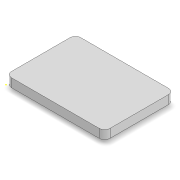
# Autodesk Inventor part: Gyro_box_Top
Saved by Autodesk Inventor 2020 (Build 240168000, 168)
## iProperties
Created: 2019-08-08
Part Number: Gyro_box_Top
Material: Generic
Document SubType Name: Modeling
Designer: chitl
Density: 1 g/cm^3
Appearance: Default
Author: chitl
Autodesk Inventor part; units mm, degrees
ref_plane "YZ Plane" through (0, 0, 0) normal (1, 0, 0) x (0, 1, 0)
ref_plane "XZ Plane" through (0, 0, 0) normal (0, 1, 0) x (-1, 0, 0)
ref_plane "XY Plane" through (0, 0, 0) normal (0, 0, 1) x (1, 0, 0)
sketch "Sketch1" plane through (0, 0, 0) normal (0, 1, 0) x (-1, 0, 0)
  line L0 (0, 0) -> (-56.9976, 0)
  line L1 (-56.9976, 0) -> (-56.9976, -40.1066)
  line L2 (-56.9976, -40.1066) -> (0, -40.1066)
  line L3 (0, -40.1066) -> (0, 0)
  dimension "d0" = 40.1066
  dimension "d1" = 56.9976
  constraints: 8 end point, 2 parallel, 1 horizontal, 1 perpendicular
  measures "d0" distance of L2.end L0.start
  measures "d1" distance between parallel lines of L1 L3
extrude "Extrusion1" add sketch "Sketch1" along normal blind 5
fillet "Fillet1" radius 3.175 2 edges at (0, 2.5, 0) (0, 2.5, -40.1066)
fillet "Fillet2" radius 3.175 2 edges at (56.9976, 2.5, 0) (56.9976, 2.5, -40.1066)
sketch "Sketch2" plane through (0, 0, 0) normal (0, -1, 0) x (1, 0, 0)
  point P0 (0, 0)
sketch "Sketch3" plane through (0, 0, 0) normal (0, -1, 0) x (1, 0, 0)
  arc A0 (53.8226, -40.1066) -> (56.9976, -36.9316) centre (53.8226, -36.9316) ccw projected
  line L0 (56.9976, -3.175) -> (56.9976, -36.9316) projected
  arc A1 (56.9976, -3.175) -> (53.8226, 0) centre (53.8226, -3.175) ccw projected
  line L1 (3.175, 0) -> (53.8226, 0) projected
  arc A2 (3.175, 0) -> (0, -3.175) centre (3.175, -3.175) ccw projected
  line L2 (0, -36.9316) -> (0, -3.175) projected
  arc A3 (0, -36.9316) -> (3.175, -40.1066) centre (3.175, -36.9316) ccw projected
  line L3 (53.8226, -40.1066) -> (3.175, -40.1066) projected
  arc A4 (53.8734, -3.175) -> (53.8226, -3.1242) centre (53.8226, -3.175) ccw
  line L4 (53.8734, -3.175) -> (53.8734, -36.9316)
  arc A5 (53.8226, -36.9824) -> (53.8734, -36.9316) centre (53.8226, -36.9316) ccw
  line L5 (53.8226, -36.9824) -> (3.175, -36.9824)
  arc A6 (3.1242, -36.9316) -> (3.175, -36.9824) centre (3.175, -36.9316) ccw
  line L6 (3.1242, -36.9316) -> (3.1242, -3.175)
  arc A7 (3.175, -3.1242) -> (3.1242, -3.175) centre (3.175, -3.175) ccw
  line L7 (3.175, -3.1242) -> (53.8226, -3.1242)
  point P0 (0, 0)
  dimension "d6" = 3.1242
  constraints: 8 end point, 8 point on circle, 4 centre point, 7 other
  measures "d6" distance between parallel lines of L1 L7
extrude "Extrusion2" add sketch "Sketch3" along normal blind 2 contours L4 A5 L5 A6 L6 A7 L7 A4
body "Solid1"
